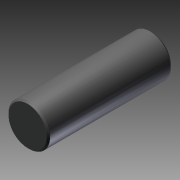
# Autodesk Inventor part: D-51
Saved by Autodesk Inventor 2011 SP1 (Build 150282100, 282)
## iProperties
Created: 2016-11-05
Part Number: D-51
Catalog Web Link: www.cadenas.de
Description: Pin-Original Line - Standard Air Cylinders
Vendor: BIMBA
Document SubType Name: Modeling
Designer: psAdmin
Manufacturer: BIMBA
Mass: 0.60147 g
Surface Area: 4.36028 cm^2
Volume: 0.60147 cm^3
Density: 1 g/cm^3
Category: PARTsolutions
Company: BIMBA
Title: D-51
Author: Cadenas PARTsolutions
Comments: Original Line - Standard Air Cylinders
PSOL_IDENT_0: {$CADENAS_DATA\23d-libs\bimba\bimba\bimba_imperial\bimba_full_line\original_line_cylinders\standard_
PSOL_IDENT_1: air_cylinders\pin.prj},147 {VTYP=3D},{NB=D-51},{LINA=D-51},{NN=Pin},{DATE=22.09.2016 13:52:24},{GEOM
PSOL_IDENT_2: DATE=15.02.2011 00:00:00},{VERSION=},{LINEID=10},{LINESUBID=-1},{WBVAR=}  {NB=D-51},{LINA=D-51},{KT=
PSOL_IDENT_3: DUMMY},{PN=D-51},{DIA=0.25000},{L=0.7500}
NN: Pin
NT: Original Line - Standard Air Cylinders
NB: D-51
NBSYN: $PN.
LINA: D-51
PN: D-51
DIA: 0.25000
L: 0.7500
SUPPLIER: BIMBA
ARTICLENO: D-51
BOMINFO: D-51
CREATOR: CADENAS GmbH
Autodesk Inventor part; units mm, degrees
ref_plane "YZ Plane" through (0, 0, 0) normal (1, 0, 0) x (0, 1, 0)
ref_plane "XZ Plane" through (0, 0, 0) normal (0, 1, 0) x (-1, 0, 0)
ref_plane "XY Plane" through (0, 0, 0) normal (0, 0, 1) x (1, 0, 0)
sketch "Sketch_1" plane through (0, 0, 0) normal (1, 0, 0) x (0, 1, 0)
  line L0 (0, -9.525) -> (0, 9.525)
  line L1 (0, 9.525) -> (2.9236, 9.525)
  line L2 (2.9236, 9.525) -> (3.175, 9.2736)
  line L3 (3.175, 9.2736) -> (3.175, -9.1694)
  line L4 (3.175, -9.1694) -> (2.8194, -9.525)
  line L5 (2.8194, -9.525) -> (0, -9.525)
  line L6 (0, -9.525) -> (0, 9.525)
  constraints: 14 end point
revolve "Revolution1" add sketch "Sketch_1" angle 360 about axis through (0, 0, -9.525) along (0, 0, -1)
ref_plane "dia1_XY" through (-3.175, 0, 0) normal (0, 0, 1) x (1, 0, 0)
ref_plane "dia1_YZ" through (-3.175, 0, 0) normal (1, 0, 0) x (0, 1, 0)
ref_plane "dia1_ZX" through (-3.175, 0, 0) normal (0, 1, 0) x (0, 0, 1)
ref_plane "dia2_XY" through (3.175, 0, 0) normal (0, 0, 1) x (1, 0, 0)
ref_plane "dia2_YZ" through (3.175, 0, 0) normal (1, 0, 0) x (0, 1, 0)
ref_plane "dia2_ZX" through (3.175, 0, 0) normal (0, 1, 0) x (0, 0, 1)
ref_plane "pin_XY" through (0, 0, 0) normal (0, 0, 1) x (1, 0, 0)
ref_plane "pin_YZ" through (0, 0, 0) normal (1, 0, 0) x (0, 1, 0)
ref_plane "pin_ZX" through (0, 0, 0) normal (0, 1, 0) x (0, 0, 1)
ref_plane "pin1_XY" through (0, 0, 9.525) normal (1, 0, 0) x (0, 0, -1)
ref_plane "pin1_YZ" through (0, 0, 9.525) normal (0, 0, -1) x (0, 1, 0)
ref_plane "pin1_ZX" through (0, 0, 9.525) normal (0, 1, 0) x (1, 0, 0)
ref_plane "pin2_XY" through (0, 0, -9.525) normal (1, 0, 0) x (0, 0, -1)
ref_plane "pin2_YZ" through (0, 0, -9.525) normal (0, 0, -1) x (0, 1, 0)
ref_plane "pin2_ZX" through (0, 0, -9.525) normal (0, 1, 0) x (1, 0, 0)
body "Solid1"
